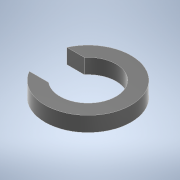
# Autodesk Inventor part: Rubberfoot
Saved by Autodesk Inventor 2022 (Build 260153000, 153)
## iProperties
Created: 2021-11-22
Part Number: Rubberfoot
Material: Caucho, Silicona
Document SubType Name: Modeling
Designer: JK
Density: 1.25 g/cm^3
Appearance: Suave - Negro
Author: JK
Autodesk Inventor part; units mm, degrees
ref_plane "YZ Plane" through (0, 0, 0) normal (1, 0, 0) x (0, 1, 0)
ref_plane "XZ Plane" through (0, 0, 0) normal (0, 1, 0) x (-1, 0, 0)
ref_plane "XY Plane" through (0, 0, 0) normal (0, 0, 1) x (1, 0, 0)
sketch "Boceto1" plane through (0, 0, 0) normal (0, 1, 0) x (-1, 0, 0)
  circle A0 centre (0, 0) radius 5.65
  circle A1 centre (0, 0) radius 8.65
  line L0 (0, 0) -> (6.6609, -5.5186)
  line L1 (0, 0) -> (5.5186, 6.6609)
  line L2 (3.6046, 4.3508) -> (7.4762, 4.3508)
  line L3 (4.3508, -3.6046) -> (7.8632, -3.6046)
  point P0 (-0.8522, 8.6079)
  point P1 (-0.8522, -8.6079)
  point P2 (3.6046, 4.3508)
  point P3 (4.3508, -3.6046)
  dimension "d0" = 11.3
  dimension "d1" = 3
  dimension "d5" = 90
  constraints: 8 end point, 8 point on circle, 2 centre point, 2 coincident, 2 point on line, 1 horizontal, 1 parallel
  measures "d0" diameter of A0
  measures "d1" radial gap between concentric circles of A0 A1
  measures "d5" angle of L0 L1
extrude "Extrusión1" add sketch "Boceto1" along normal blind 3 contours A0 L0 A1 L1 | L1 A1 L2 | L3 A1 L0
